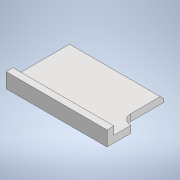
# Autodesk Inventor part: Part17
Saved by Autodesk Inventor 2022 (Build 260153000, 153)
## iProperties
Created: 2022-06-07
Part Number: Part17
Material: Generic
Document SubType Name: Modeling
Designer: tecware
Density: 1 g/cm^3
Appearance: Default
Author: tecware
## iProperties of the stored document tray_3DPrint.ipt
Created: 2022-06-07
Part Number: tray_3DPrint
Material: Generic
Document SubType Name: Modeling
Designer: tecware
Density: 1 g/cm^3
Appearance: Default
Author: tecware
Autodesk Inventor part; units mm, degrees
ref_plane "YZ Plane" through (0, 0, 0) normal (1, 0, 0) x (0, 1, 0)
ref_plane "XZ Plane" through (0, 0, 0) normal (0, 1, 0) x (-1, 0, 0)
ref_plane "XY Plane" through (0, 0, 0) normal (0, 0, 1) x (1, 0, 0)
sketch "Sketch1" plane through (0, 0, 0) normal (0, 0, 1) x (1, 0, 0)
  line L0 (0.5037, -0.606) -> (30.1037, -0.606)
  line L1 (30.1037, -0.606) -> (30.1037, -4.956)
  line L2 (30.1037, -4.956) -> (0.5037, -4.956)
  line L3 (0.5037, -4.956) -> (0.5037, -0.606)
  point P0 (0, 0)
  dimension "d1" = 4.35
  dimension "d2" = 29.6
  constraints: 8 end point, 4 parallel, 1 perpendicular
  measures "d1" distance of L2.end L0.start
  measures "d2" distance of L0.start L0.end
extrude "Extrusion1" add sketch "Sketch1" along normal blind 2
sketch "Sketch2" plane through (0, 0, 0) normal (0, 0, -1) x (-1, 0, 0)
  line L0 (-30.1037, -4.956) -> (-0.5037, -4.956)
  line L1 (-0.5037, -4.956) -> (-0.5037, -2.956)
  line L2 (-0.5037, -2.956) -> (-30.1037, -2.956)
  line L3 (-30.1037, -2.956) -> (-30.1037, -4.956)
  line L4 (-0.5037, -4.956) -> (-30.1037, -4.956) projected
  line L5 (-30.1037, -4.956) -> (-30.1037, -0.606) projected
  dimension "d11" = 29.6
  dimension "d12" = 2
  constraints: 8 end point, 2 collinear, 2 perpendicular
  measures "d11" distance of L2.end L1.end
  measures "d12" distance of L1.end L0.end
extrude "Extrusion2" add sketch "Sketch2" along normal blind 17.6
chamfer "Chamfer2" distance 1 angle 45 1 edges at (15.3037, -2.956, -17.6)
sketch "Sketch3" plane through (0.5037, -2.956, 0) normal (0, 1, 0) x (1, 0, 0)
  line L0 (29.6, 17.6) -> (0, 17.6) projected
  line L1 (29.6, 17.6) -> (26.6, 17.6)
  line L2 (26.6, 17.6) -> (26.6, 5)
  line L3 (26.6, 5) -> (29.6, 5)
  line L4 (29.6, 5) -> (29.6, 17.6)
  point P0 (-0.5037, 0)
  dimension "d16" = 3
  dimension "d17" = 12.6
  constraints: 8 end point
  measures "d16" distance of L3.end L2.end
  measures "d17" distance of L2.end L1.end
extrude "Extrusion3" cut sketch "Sketch3" against normal through all
fillet "Fillet1" radius 3 1 edges at (27.1037, -3.956, -5)
body "Solid1"
